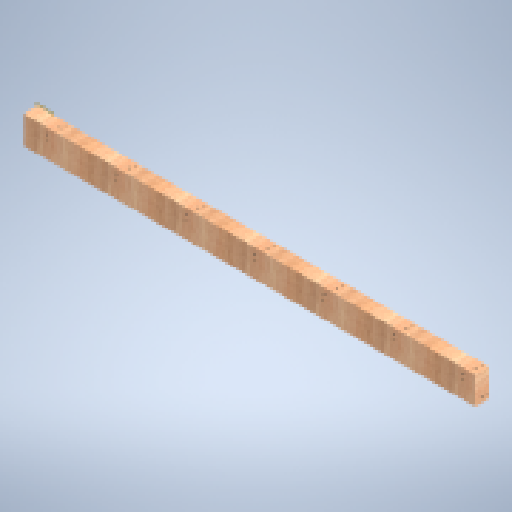
# Autodesk Inventor part: 2X4X65.191
Saved by Autodesk Inventor 2025 (Build 290162000, 162)
## iProperties
Created: 2024-09-08
Part Number: 2X4X65.191
Material: Wood (Birch)
Document SubType Name: Modeling
Designer: Win
Density: 0.55 g/cm^3
Appearance: Birch - Natural Polished
Author: Win
Autodesk Inventor part; units mm, degrees
ref_plane "YZ Plane" through (0, 0, 0) normal (1, 0, 0) x (0, 1, 0)
ref_plane "XZ Plane" through (0, 0, 0) normal (0, 1, 0) x (-1, 0, 0)
ref_plane "XY Plane" through (0, 0, 0) normal (0, 0, 1) x (1, 0, 0)
ref_plane "Work Plane1" through (0, 0, 0) normal (0, 0, 1) x (1, 0, 0)
sketch "Sketch1" plane through (0, 0, 0) normal (0, 0, 1) x (1, 0, 0)
  line L0 (-55.6518, 0) -> (0, 0) projected
  line L1 (-55.6518, 0) -> (-55.6518, -101.6) projected
  line L2 (0, -101.6) -> (-55.6518, -101.6) projected
  line L3 (0, 0) -> (0, -101.6) projected
  line L4 (1549.4, -50.8) -> (1651, -50.8) projected
  line L5 (1651, -50.8) -> (1651, 0) projected
  line L6 (1549.4, 0) -> (1651, 0) projected
  line L7 (1549.4, -50.8) -> (1549.4, 0) projected
  line L8 (-55.6518, -101.6) -> (1600.2, -101.6)
  line L9 (1600.2, -101.6) -> (1600.2, 0)
  line L10 (1600.2, 0) -> (-55.6518, 0)
  line L11 (-55.6518, 0) -> (-55.6518, -101.6)
  point P0 (0, 0)
  constraints: 8 end point, 2 parallel, 1 horizontal, 1 midpoint, 1 perpendicular
extrude "Extrusion1" add sketch "Sketch1" along normal blind 50.8 contours L0 L3 L2 L1 | L10 L7 L4 L9 L8 L3 | L6 L9 L4 L7
sketch "Sketch3" plane through (-55.6518, -101.6, 0) normal (0, -1, 0) x (1, 0, 0)
  line L0 (0, 0) -> (101.6, 0) projected
  line L1 (101.6, 0) -> (1270, 1117.6) projected
  line L2 (1270, 1117.6) -> (1270, 1219.2) projected
  line L3 (1270, 1219.2) -> (0, 0) projected
  line L4 (0, 0) -> (101.6, 0) projected
  line L5 (101.6, 0) -> (1270, 1117.6) projected
  line L6 (1270, 1117.6) -> (1270, 1219.2) projected
  line L7 (1270, 1219.2) -> (0, 0) projected
  line L8 (0, 0) -> (0, 50.8) projected
  line L9 (0, 0) -> (0, 50.8)
  line L10 (0, 50.8) -> (52.9167, 50.8)
  line L11 (0, 50.8) -> (1655.8518, 50.8) projected
  line L12 (0, 0) -> (1655.8518, 0) projected
  line L13 (52.9167, 50.8) -> (0, 0)
  point P0 (55.6518, 0)
  point P1 (52.9167, 50.8)
  constraints: 6 end point, 2 collinear, 2 point on line
extrude "Extrusion3" cut sketch "Sketch3" against normal blind 101.6 contours L8 L10 L3
ref_plane "Work Plane2" through (1620.7482, -50.8, -965.2) normal (0, 1, 0) x (0, 0, -1)
sketch "Sketch4" plane through (1600.2, 0, 50.8) normal (0, 1, 0) x (1, 0, 0)
  line L0 (-30.2518, 1981.2) -> (-30.2518, 50.8) projected
  line L1 (-30.2518, 50.8) -> (71.3482, 50.8) projected
  line L2 (71.3482, 50.8) -> (71.3482, 1981.2) projected
  line L3 (71.3482, 1981.2) -> (-30.2518, 1981.2) projected
  line L4 (-30.2518, 1981.2) -> (-30.2518, 50.8) projected
  line L5 (-30.2518, 50.8) -> (71.3482, 50.8) projected
  line L6 (71.3482, 50.8) -> (71.3482, 1981.2) projected
  line L7 (71.3482, 1981.2) -> (-30.2518, 1981.2) projected
  line L8 (20.5482, 50.8) -> (0, 50.8)
  line L9 (-1602.9352, 0) -> (0, 0) projected
  line L10 (0, 50.8) -> (0, 0)
  line L11 (0, 0) -> (20.5482, 0)
  line L12 (20.5482, 0) -> (20.5482, 50.8)
  point P0 (-1600.2, 50.8)
  point P1 (20.5482, 50.8)
  constraints: 8 end point, 3 perpendicular, 1 collinear, 1 midpoint
extrude "Extrusion4" add sketch "Sketch4" against normal blind 101.6 contours L1 L12 L11 L10
body "Solid1"
